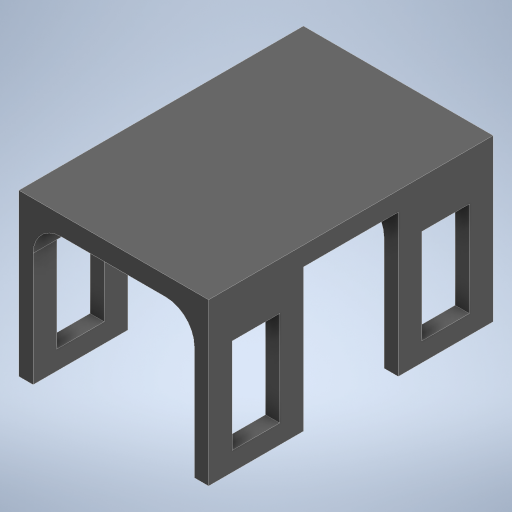
# Autodesk Inventor part: connetcor_female
Saved by Autodesk Inventor 2024.1 (Build 281209000, 209)
## iProperties
Created: 2025-09-28
Part Number: connetcor_female
Material: 一般
Document SubType Name: Modeling
Designer: hibik
Density: 1 g/cm^3
Appearance: 既定
Author: hibik
Autodesk Inventor part; units mm, degrees
ref_plane "YZ Plane" through (0, 0, 0) normal (1, 0, 0) x (0, 1, 0)
ref_plane "XZ Plane" through (0, 0, 0) normal (0, 1, 0) x (-1, 0, 0)
ref_plane "XY Plane" through (0, 0, 0) normal (0, 0, 1) x (1, 0, 0)
sketch "スケッチ1" plane through (0, 0, 0) normal (0, 0, 1) x (1, 0, 0)
  line L0 (-10, 17) -> (0, 17)
  line L1 (0, 17) -> (0, 15)
  line L2 (0, 15) -> (-10, 15)
  line L3 (-10, 15) -> (-10, 17)
  line L4 (0, -3.4) -> (0, 20.4) projected
  point P0 (0, 0)
  dimension "d0" = 10
  dimension "d1" = 2
  dimension "d2" = 15
  constraints: 8 end point, 2 parallel, 1 collinear, 1 horizontal, 1 perpendicular
  measures "d0" distance of L0.start L0.end
  measures "d1" distance of L2.end L0.start
  measures "d2" distance from line of point (0, 0) L2
extrude "押し出し1" add sketch "スケッチ1" along normal blind 5
sketch "スケッチ2" plane through (0, 0, 5) normal (0, 0, 1) x (1, 0, 0)
  line L0 (0, 17) -> (-10, 17) projected
  line L1 (-10, 17) -> (-8.5, 17)
  line L2 (-8.5, 17) -> (-8.5, 0)
  line L3 (-8.5, 0) -> (-10, 0)
  line L4 (-10, 0) -> (-10, 17)
  line L5 (-10, 15) -> (0, 15) projected
  line L6 (0, 15) -> (0, 17) projected
  line L7 (0, 17) -> (-10, 17) projected
  line L8 (-10, 17) -> (-10, 15) projected
  point P0 (0, 0)
  point P1 (-8.5, 15)
  dimension "d5" = 1.5
  constraints: 8 end point, 2 parallel, 1 horizontal, 1 perpendicular, 1 point on line
  measures "d5" distance of L2.end L3.end
extrude "押し出し2" add sketch "スケッチ2" along normal blind 10
sketch "スケッチ3" plane through (-8.5, 0, 5) normal (1, 0, 0) x (0, 0, -1)
  line L0 (-7.5, 12) -> (-2.5, 12)
  line L1 (-2.5, 12) -> (-2.5, 2)
  line L2 (-2.5, 2) -> (-7.5, 2)
  line L3 (-7.5, 2) -> (-7.5, 12)
  line L4 (0, 0) -> (-10, 0) projected
  line L5 (0, 15) -> (-10, 15) projected
  point P0 (5, 0)
  point P1 (-5, 2)
  point P2 (-5, 0)
  dimension "d8" = 2
  dimension "d9" = 5
  dimension "d13" = 3
  constraints: 8 end point, 2 midpoint, 2 parallel, 1 horizontal, 1 perpendicular, 1 vertical alignment
  measures "d8" distance between parallel lines of L4 L2
  measures "d9" distance of L1.end L2.end
  measures "d13" distance between parallel lines of L5 L0
extrude "押し出し3" cut sketch "スケッチ3" against normal through all
fillet "フィレット1" radius 3 1 edges at (-8.5, 15, 10)
mirror "ミラー1" about plane through (0, 15, 0) normal (1, 0, 0)
mirror "ミラー2" about plane through (-5, 16, 0) normal (0, 0, -1)
